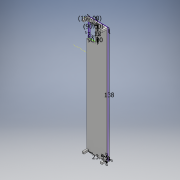
# Autodesk Inventor part: case-top
Saved by Autodesk Inventor 2017 (Build 210142000, 142)
## iProperties
Created: 2026-06-28
Part Number: case-top
Material: Generic
Document SubType Name: Modeling
Designer: hashire umamusume
Density: 1 g/cm^3
Appearance: Default
Author: hashire umamusume
Autodesk Inventor part; units mm, degrees
ref_plane "YZ Plane" through (0, 0, 0) normal (1, 0, 0) x (0, 1, 0)
ref_plane "XZ Plane" through (0, 0, 0) normal (0, 1, 0) x (-1, 0, 0)
ref_plane "XY Plane" through (0, 0, 0) normal (0, 0, 1) x (1, 0, 0)
sketch "Sketch1" plane through (0, 0, 0) normal (0, 1, 0) x (-1, 0, 0)
  line L0 (0, 0) -> (-23.5, 0)
  line L1 (-23.5, 0) -> (-23.5, -138)
  line L2 (-23.5, -138) -> (0, -138)
  line L3 (0, -138) -> (0, 0)
  line L4 (-2, -2) -> (-21.5, -2)
  line L5 (-21.5, -2) -> (-21.5, -136)
  line L6 (-21.5, -136) -> (-2, -136)
  line L7 (-2, -136) -> (-2, -2)
  line L8 (-2, -2) -> (0, -2)
  line L9 (0, -2) -> (0, 0)
  line L10 (0, 0) -> (-2, 0)
  line L11 (-2, 0) -> (-2, -2)
  line L12 (-21.5, -2) -> (-23.5, -2)
  line L13 (-23.5, -2) -> (-23.5, 0)
  line L14 (-23.5, 0) -> (-21.5, 0)
  line L15 (-21.5, 0) -> (-21.5, -2)
  line L16 (-21.5, -136) -> (-23.5, -136)
  line L17 (-23.5, -136) -> (-23.5, -138)
  line L18 (-23.5, -138) -> (-21.5, -138)
  line L19 (-21.5, -138) -> (-21.5, -136)
  line L20 (-2, -136) -> (0, -136)
  line L21 (0, -136) -> (0, -138)
  line L22 (0, -138) -> (-2, -138)
  line L23 (-2, -138) -> (-2, -136)
  line L24 (-2, -38.4581) -> (17.5, -38.4581) construction
  line L25 (-21.5, -24) -> (-2, -24)
  line L26 (-2, -4.3088) -> (-10, -4.3088)
  line L27 (-2, -4.3088) -> (6, -4.3088) construction
  line L28 (-10, -4.3088) -> (-10, -22.3088)
  line L29 (-10, -22.3088) -> (-2, -22.3088)
  line L30 (-2, -4.3088) -> (0, -4.3088)
  line L31 (0, -4.3088) -> (0, -22.3088)
  line L32 (0, -22.3088) -> (-2, -22.3088)
  line L33 (-2, -22.3088) -> (-2, -4.3088)
  dimension "d0" = 23.5
  dimension "d1" = 138
  dimension "d2" = 2
  dimension "d3" = 2
  dimension "d5" = 2
  dimension "d6" = 2
  dimension "d8" = 22
  dimension "d24" = 8
  dimension "d25" = 180
  dimension "d26" = 18
  dimension "d27" = 90
  dimension "d28" = 90
  constraints: 68 end point, 14 parallel, 10 horizontal, 9 perpendicular, 6 point on line, 1 collinear
  measures "d0" distance of L2.end L1.end
  measures "d1" distance of L1.end L0.end
  measures "d2" distance between parallel lines of L2 L6
  measures "d3" distance between parallel lines of L5 L1
  measures "d5" distance between parallel lines of L0 L4
  measures "d6" distance between parallel lines of L3 L7
  measures "d8" distance between parallel lines of L4 L25
  measures "d24" distance of L26.start L26.end
  measures "d25" angle of L26 L27
  measures "d26" distance of L26.end L28.end
  measures "d27" angle of L28 L26
  measures "d28" angle of L29 L28
extrude "Extrusion1" add sketch "Sketch1" against normal blind 1.6
extrude "Extrusion2" add sketch "Sketch1" against normal blind 7 contours L3 L8 L11 L0 | L15 L12 L1 L0 | L3 L2 L23 L20 | L16 L19 L2 L1
extrude "Extrusion4" cut sketch "Sketch1" against normal blind 3 contours L3 L32 L7 L30 | L7 L29 L28 L26
body "Solid1"
